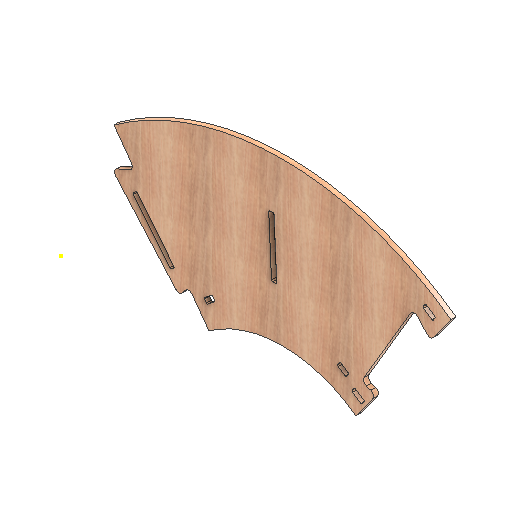
# Autodesk Inventor part: Platform B3
Saved by Autodesk Inventor 2021 (Build 250183000, 183)
## iProperties
Created: 2020-05-09
Part Number: Platform B3
Material: Wood (Birch)
Document SubType Name: Modeling
Designer: Dan Wikman
Density: 0.55 g/cm^3
Appearance: Birch - Natural Polished
Mass: 5234.7 g
Surface Area: 11417.5 cm^2
Volume: 9517.64 cm^3
Autodesk Inventor part; units mm, degrees
ref_plane "YZ Plane" through (0, 0, 0) normal (1, 0, 0) x (0, 1, 0)
ref_plane "XZ Plane" through (0, 0, 0) normal (0, 1, 0) x (-1, 0, 0)
ref_plane "XY Plane" through (0, 0, 0) normal (0, 0, 1) x (1, 0, 0)
sketch "Sketch1" plane through (0, 0, 0) normal (0, 0, 1) x (1, 0, 0)
  point P0 (0, 0)
sketch "CONTOURS" plane through (0, 0, 0) normal (0, 0, 1) x (1, 0, 0)
  arc A0 (1138.7708, 133.0427) -> (1131.5929, 155.3323) centre (1127.04, 141.5656) ccw
  line L0 (1131.5929, 155.3323) -> (1115.5781, 160.6286)
  arc A1 (1107.0938, 183.2185) -> (1115.5781, 160.6286) centre (1120.445, 175.3447) ccw
  line L1 (1107.0938, 183.2185) -> (1274.33, 466.7921)
  arc A2 (1299.254, 469.2294) -> (1274.33, 466.7921) centre (1287.6812, 458.9183) ccw
  line L2 (1299.254, 469.2294) -> (1333.4216, 430.8808)
  arc A3 (1333.4216, 430.8808) -> (1355.9785, 432.0038) centre (1344.2478, 440.5267) ccw
  line L3 (1355.9785, 432.0038) -> (1419.4157, 519.3176)
  arc A4 (1419.4157, 519.3176) -> (208.109, 519.3881) centre (813.7138, -315.0977) ccw
  line L4 (208.109, 519.3881) -> (271.5978, 432.0034)
  arc A5 (265.2883, 408.6999) -> (271.5978, 432.0034) centre (259.0581, 422.8927) ccw
  line L5 (265.2883, 408.6999) -> (218.2583, 388.055)
  arc A6 (218.2583, 388.055) -> (213.2217, 365.1756) centre (224.0866, 374.778) ccw
  line L6 (213.2217, 365.1756) -> (431.2374, 118.4955)
  arc A7 (431.2374, 118.4955) -> (453.7882, 119.5137) centre (442.1023, 128.0978) ccw
  line L7 (453.7882, 119.5137) -> (463.7742, 133.108)
  arc A8 (488.8058, 133.0425) -> (463.7742, 133.108) centre (476.2661, 123.9318) ccw
  line L8 (488.8058, 133.0425) -> (549.6876, 49.246)
  arc A9 (1077.8891, 49.2462) -> (549.6876, 49.246) centre (813.7885, -315.108) ccw
  line L9 (1077.8891, 49.2462) -> (1138.7708, 133.0427)
  constraints: 20 end point, 20 point on circle, 10 centre point
sketch "HOLES" plane through (0, 0, 0) normal (0, 0, 1) x (1, 0, 0)
  line L0 (287.205, 350.9682) -> (278.6203, 344.0905)
  arc A0 (278.6203, 344.0905) -> (277.9995, 338.4678) centre (281.1212, 340.9688) ccw
  line L1 (277.9995, 338.4678) -> (408.6757, 175.3582)
  arc A1 (408.6757, 175.3582) -> (414.2984, 174.7375) centre (411.7974, 177.8592) ccw
  line L2 (414.2984, 174.7375) -> (422.8831, 181.6152)
  arc A2 (422.8831, 181.6152) -> (423.5039, 187.2379) centre (420.3822, 184.7369) ccw
  line L3 (423.5039, 187.2379) -> (292.8277, 350.3475)
  arc A3 (292.8277, 350.3475) -> (287.205, 350.9682) centre (289.706, 347.8465) ccw
  arc A4 (783.5127, 529.4978) -> (779.3287, 533.3049) centre (779.5172, 529.3094) ccw
  line L4 (783.5127, 529.4978) -> (793.3586, 320.7299)
  arc A5 (789.5515, 316.5459) -> (793.3586, 320.7299) centre (789.363, 320.5414) ccw
  line L5 (789.5515, 316.5459) -> (778.5637, 316.0277)
  arc A6 (774.3797, 319.8348) -> (778.5637, 316.0277) centre (778.3752, 320.0232) ccw
  line L6 (774.3797, 319.8348) -> (764.5338, 528.6027)
  arc A7 (768.3409, 532.7867) -> (764.5338, 528.6027) centre (768.5294, 528.7912) ccw
  line L7 (768.3409, 532.7867) -> (779.3287, 533.3049)
  line L8 (569.7888, 155.0903) -> (562.9111, 163.675)
  arc A8 (562.9111, 163.675) -> (557.2884, 164.2957) centre (559.7894, 161.174) ccw
  line L9 (557.2884, 164.2957) -> (533.8755, 145.5384)
  arc A9 (533.8755, 145.5384) -> (533.2548, 139.9157) centre (536.3765, 142.4167) ccw
  line L10 (533.2548, 139.9157) -> (540.1325, 131.331)
  arc A10 (540.1325, 131.331) -> (545.7552, 130.7102) centre (543.2542, 133.832) ccw
  line L11 (545.7552, 130.7102) -> (569.168, 149.4676)
  arc A11 (569.168, 149.4676) -> (569.7888, 155.0903) centre (566.6671, 152.5893) ccw
  line L12 (1012.5411, 175.9713) -> (1018.5803, 185.1652)
  arc A12 (1024.1197, 186.3123) -> (1018.5803, 185.1652) centre (1021.9236, 182.9691) ccw
  line L13 (1024.1197, 186.3123) -> (1049.1939, 169.8417)
  arc A13 (1050.3411, 164.3024) -> (1049.1939, 169.8417) centre (1046.9978, 166.4985) ccw
  line L14 (1059.1699, 932.849) -> (1052.9484, 923.7775)
  arc A14 (1047.3873, 922.7411) -> (1052.9484, 923.7775) centre (1049.6497, 926.0399) ccw
  line L15 (1047.3873, 922.7411) -> (1017.6987, 943.1026)
  arc A15 (1016.6623, 948.6637) -> (1017.6987, 943.1026) centre (1019.9611, 946.4013) ccw
  line L16 (1016.6623, 948.6637) -> (1022.8839, 957.7352)
  arc A16 (1028.445, 958.7715) -> (1022.8839, 957.7352) centre (1026.1826, 955.4728) ccw
  line L17 (1028.445, 958.7715) -> (1058.1336, 938.4101)
  arc A17 (1059.1699, 932.849) -> (1058.1336, 938.4101) centre (1055.8712, 935.1114) ccw
  arc A18 (2370.6146, 1037.7855) -> (2376.2246, 1037.059) centre (2373.7829, 1040.2273) ccw
  line L18 (2370.6146, 1037.7855) -> (2296.1408, 1134.417)
  arc A19 (2296.8672, 1140.027) -> (2296.1408, 1134.417) centre (2299.309, 1136.8588) ccw
  line L19 (2296.8672, 1140.027) -> (2305.5799, 1146.7419)
  arc A20 (2311.1899, 1146.0154) -> (2305.5799, 1146.7419) centre (2308.0217, 1143.5736) ccw
  line L20 (2311.1899, 1146.0154) -> (2385.6638, 1049.3839)
  arc A21 (2384.9373, 1043.7739) -> (2385.6638, 1049.3839) centre (2382.4955, 1046.9421) ccw
  line L21 (2384.9373, 1043.7739) -> (2376.2246, 1037.059)
  line L22 (1175.8209, 1180.7295) -> (1169.5993, 1171.658)
  arc A22 (1169.5993, 1171.658) -> (1170.6357, 1166.0969) centre (1172.898, 1169.3956) ccw
  line L23 (1170.6357, 1166.0969) -> (1200.3242, 1145.7355)
  arc A23 (1200.3242, 1145.7355) -> (1205.8854, 1146.7718) centre (1202.5866, 1149.0342) ccw
  line L24 (1205.8854, 1146.7718) -> (1212.1069, 1155.8433)
  arc A24 (1212.1069, 1155.8433) -> (1211.0706, 1161.4044) centre (1208.8082, 1158.1057) ccw
  line L25 (1211.0706, 1161.4044) -> (1181.382, 1181.7659)
  arc A25 (1181.382, 1181.7659) -> (1175.8209, 1180.7295) centre (1179.1196, 1178.4671) ccw
  line L26 (1050.3411, 164.3024) -> (1044.3019, 155.1085)
  arc A26 (1038.7625, 153.9613) -> (1044.3019, 155.1085) centre (1040.9586, 157.3046) ccw
  line L27 (1038.7625, 153.9613) -> (1013.6883, 170.4319)
  arc A27 (1012.5411, 175.9713) -> (1013.6883, 170.4319) centre (1015.8843, 173.7752) ccw
  line L28 (1101.0619, 97.7126) -> (1107.1011, 106.9065)
  arc A28 (1107.1011, 106.9065) -> (1105.954, 112.4458) centre (1103.7579, 109.1026) ccw
  line L29 (1105.954, 112.4458) -> (1075.8649, 132.2106)
  arc A29 (1075.8649, 132.2106) -> (1070.3255, 131.0634) centre (1073.6688, 128.8673) ccw
  line L30 (1070.3255, 131.0634) -> (1064.2863, 121.8695)
  arc A30 (1064.2863, 121.8695) -> (1065.4335, 116.3302) centre (1067.6295, 119.6734) ccw
  line L31 (1065.4335, 116.3302) -> (1095.5226, 96.5655)
  arc A31 (1095.5226, 96.5655) -> (1101.0619, 97.7126) centre (1097.7187, 99.9087) ccw
  line L32 (1362.3431, 495.4778) -> (1356.3039, 486.2839)
  arc A32 (1350.7646, 485.1368) -> (1356.3039, 486.2839) centre (1352.9607, 488.48) ccw
  line L33 (1350.7646, 485.1368) -> (1320.6755, 504.9015)
  arc A33 (1319.5283, 510.4408) -> (1320.6755, 504.9015) centre (1322.8716, 508.2448) ccw
  line L34 (1319.5283, 510.4408) -> (1325.5675, 519.6347)
  arc A34 (1331.1069, 520.7819) -> (1325.5675, 519.6347) centre (1328.9108, 517.4387) ccw
  line L35 (1331.1069, 520.7819) -> (1361.196, 501.0172)
  arc A35 (1362.3431, 495.4778) -> (1361.196, 501.0172) centre (1358.9999, 497.6739) ccw
  line L36 (1264.9795, 244.1751) -> (1271.0187, 253.369)
  arc A36 (1276.558, 254.5161) -> (1271.0187, 253.369) centre (1274.3619, 251.1729) ccw
  line L37 (1276.558, 254.5161) -> (1306.6471, 234.7514)
  arc A37 (1307.7943, 229.2121) -> (1306.6471, 234.7514) centre (1304.451, 231.4082) ccw
  line L38 (1307.7943, 229.2121) -> (1301.7551, 220.0182)
  arc A38 (1296.2157, 218.871) -> (1301.7551, 220.0182) centre (1298.4118, 222.2143) ccw
  line L39 (1296.2157, 218.871) -> (1266.1266, 238.6358)
  arc A39 (1264.9795, 244.1751) -> (1266.1266, 238.6358) centre (1268.3227, 241.979) ccw
  line L40 (1526.2607, 641.9403) -> (1520.2215, 632.7464)
  arc A40 (1520.2215, 632.7464) -> (1521.3686, 627.2071) centre (1523.5647, 630.5503) ccw
  line L41 (1521.3686, 627.2071) -> (1551.4577, 607.4424)
  arc A41 (1551.4577, 607.4424) -> (1556.9971, 608.5895) centre (1553.6538, 610.7856) ccw
  line L42 (1556.9971, 608.5895) -> (1563.0363, 617.7834)
  arc A42 (1563.0363, 617.7834) -> (1561.8891, 623.3227) centre (1559.6931, 619.9795) ccw
  line L43 (1561.8891, 623.3227) -> (1531.8, 643.0875)
  arc A43 (1531.8, 643.0875) -> (1526.2607, 641.9403) centre (1529.6039, 639.7442) ccw
  constraints: 88 end point, 88 point on circle, 44 centre point
sketch "LETTERS" plane through (0, 0, 0) normal (0, 0, 1) x (1, 0, 0)
  arc A0 (1107.5534, 367.1718) -> (1103.7785, 359.006) centre (1105.6754, 363.0845) ccw
  line L0 (1107.5534, 367.1718) -> (1115.5892, 363.4795)
  arc A1 (1112.0249, 376.8584) -> (1107.5534, 367.1718) centre (1109.7806, 372.0191) ccw
  line L1 (1120.1257, 373.1016) -> (1112.0249, 376.8584)
  line L2 (1111.8629, 355.2459) -> (1120.1257, 373.1016)
  line L3 (1103.7785, 359.006) -> (1111.8629, 355.2459)
  constraints: 8 end point, 4 point on circle, 4 tangent, 2 centre point
extrude "Extrusion2" add sketch "CONTOURS" along normal blind 18
extrude "Extrusion3" cut sketch "HOLES" along normal through all contours A3 L3 A2 L2 A1 L1 A0 L0 | L4 A5 L5 A6 L6 A7 L7 A4 | A11 L11 A10 L10 A9 L9 A8 L8 | L12 A12 L13 A13 L26 A26 L27 A27 | A31 L31 A30 L30 A29 L29 A28 L28 | L32 A32 L33 A33 L34 A34 L35 A35
body "Solid2"
